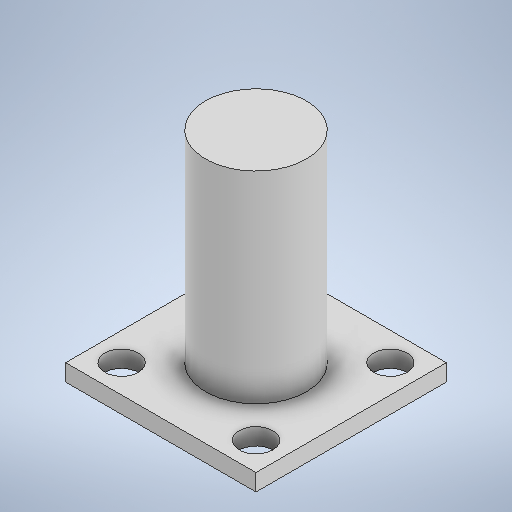
# Autodesk Inventor part: BNC connector
Saved by Autodesk Inventor 2025 (Build 290162000, 162)
## iProperties
Created: 2024-04-12
Part Number: BNC connector
Material: Generic
Document SubType Name: Modeling
Designer: mahal
Density: 1 g/cm^3
Appearance: Default
Author: mahal
Autodesk Inventor part; units mm, degrees
ref_plane "YZ Plane" through (0, 0, 0) normal (1, 0, 0) x (0, 1, 0)
ref_plane "XZ Plane" through (0, 0, 0) normal (0, 1, 0) x (-1, 0, 0)
sketch "Sketch1" plane through (0, 0, 0) normal (0, 1, 0) x (-1, 0, 0)
  line L0 (8.5, 8.5) -> (-8.5, 8.5)
  line L1 (-8.5, 8.5) -> (-8.5, -8.5)
  line L2 (-8.5, -8.5) -> (8.5, -8.5)
  line L3 (8.5, -8.5) -> (8.5, 8.5)
  line L4 (8.5, 8.5) -> (-8.5, -8.5) construction
  line L5 (-8.5, 8.5) -> (8.5, -8.5) construction
  line L6 (6, 6) -> (-6, 6)
  line L7 (-6, 6) -> (-6, -6)
  line L8 (-6, -6) -> (6, -6)
  line L9 (6, -6) -> (6, 6)
  line L10 (6, 6) -> (-6, -6) construction
  line L11 (-6, 6) -> (6, -6) construction
  circle A0 centre (6, 6) radius 1.5
  line L12 (6, 0) -> (4.5, 0)
  line L13 (0, 6) -> (0, 3.3641)
  circle A1 centre (6, -6) radius 1.5
  circle A2 centre (-6, 6) radius 1.5
  circle A3 centre (-6, -6) radius 1.5
  circle A4 centre (0, 0) radius 4.5
  dimension "d0" = 17
  dimension "d1" = 17
  dimension "d2" = 12
  dimension "d3" = 12
  dimension "d4" = 3
  dimension "d5" = 9
  constraints: 28 end point, 6 midpoint, 5 centre point, 4 parallel, 3 horizontal, 3 symmetric about line, 2 coincident, 2 perpendicular, 1 vertical, 3 other
  measures "d0" distance of L2.end L1.end
  measures "d1" distance of L1.end L0.end
  measures "d2" distance of L8.end L7.end
  measures "d3" distance of L7.end L6.end
  measures "d4" diameter of A0
  measures "d5" diameter of A4
extrude "Extrusion1" add sketch "Sketch1" along normal blind 1.5 contours L3 L2 L1 L0 | L13 A4 L12 L9 A1 L8 A3 L7 A2 L6 | L6 A0 L9 L12 A4 L13 | A4
ref_plane "Work Plane1" through (0, 1.5, 0) normal (0, 1, 0) x (1, 0, 0)
sketch "Sketch2" plane through (0, 1.5, 0) normal (0, 1, 0) x (1, 0, 0)
  circle A0 centre (0, 0) radius 4.5
  dimension "d9" = 9
  constraints: 1 centre point, 1 coincident
  measures "d9" diameter of A0
extrude "Extrusion2" add sketch "Sketch2" along normal blind 18
body "Solid1"
